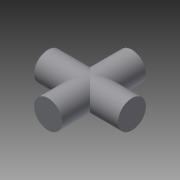
# Autodesk Inventor part: 第一次上机-示例建模
Saved by Autodesk Inventor 2013 (Build 170138000, 138)
## iProperties
Created: 2016-11-06
Part Number: 第一次上机-示例建模
Material: 常规
Document SubType Name: Modeling
Designer: Administrator
Density: 1 g/cm^3
Author: Administrator
Autodesk Inventor part; units mm, degrees
ref_plane "YZ Plane" through (0, 0, 0) normal (1, 0, 0) x (0, 1, 0)
ref_plane "XZ Plane" through (0, 0, 0) normal (0, 1, 0) x (-1, 0, 0)
ref_plane "XY Plane" through (0, 0, 0) normal (0, 0, 1) x (1, 0, 0)
sketch "草图1" plane through (0, 0, 0) normal (1, 0, 0) x (0, 1, 0)
  circle A0 centre (0, 0) radius 12.5
  dimension "d0" = 25
  constraints: 1 centre point, 1 coincident
  measures "d0" diameter of A0
extrude "拉伸1" add sketch "草图1" along normal blind 75
sketch "草图2" plane through (0, 0, 0) normal (0, 1, 0) x (-1, 0, 0)
  circle A0 centre (-37.5, 0) radius 12.5
  line L0 (0, 12.5) -> (-75, 12.5) projected
  line L1 (0, -12.5) -> (-75, -12.5) projected
  point P0 (0, 0)
  point P1 (-37.5, -12.5)
  constraints: 2 tangent, 1 centre point, 1 midpoint, 1 vertical alignment
extrude "拉伸2" add sketch "草图2" along normal mid plane 75
